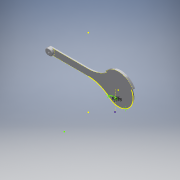
# Autodesk Inventor part: Trap
Saved by Autodesk Inventor 2019 (Build 230136000, 136)
## iProperties
Created: 2018-12-18
Part Number: Trap
Material: ABS Plastic
Document SubType Name: Modeling
Designer: assman
Density: 1.06 g/cm^3
Appearance: Smooth - White
Author: assman
Autodesk Inventor part; units mm, degrees
ref_plane "YZ Plane" through (0, 0, 0) normal (1, 0, 0) x (0, 1, 0)
ref_plane "XZ Plane" through (0, 0, 0) normal (0, 1, 0) x (-1, 0, 0)
ref_plane "XY Plane" through (0, 0, 0) normal (0, 0, 1) x (1, 0, 0)
sketch "Sketch1" plane through (0, 0, 0) normal (0, 0, 1) x (1, 0, 0)
  line L0 (-0.1193, 0) -> (89.8393, 0) construction
  line L1 (52.5778, -17.0836) -> (118.1369, -38.385) construction
  line L2 (85.3573, -27.7343) -> (99.4539, 15.6504) construction
  line L3 (-0.1193, 0) -> (89.8393, 0) construction
  circle A0 centre (-0.1193, 0) radius 89.8635 construction
  circle A1 centre (85.3573, -27.7343) radius 17.272 construction
  spline S0 degree 3 poles (0.7787, 2.3967) (0.465, 2.4986) (0.1311, 2.5381) (-0.1977, 2.5122) (-0.5266, 2.4864) (-0.8501, 2.3951) (-1.1441, 2.2453) (-1.438, 2.0956) (-1.702, 1.8874) (-1.9162, 1.6366) (-2.1305, 1.3858) (-2.2947, 1.0924) (-2.3967, 0.7787) (-2.4986, 0.465) (-2.5381, 0.1311) (-2.5122, -0.1977) (-2.4864, -0.5266) (-2.3951, -0.8501) (-2.2453, -1.1441) (-2.0956, -1.438) (-1.8874, -1.702) (-1.6366, -1.9162) (-1.3858, -2.1305) (-1.0924, -2.2947) (-0.7787, -2.3967) (-0.465, -2.4986) (-0.1311, -2.5381) (0.1977, -2.5122) (0.5266, -2.4864) (0.8501, -2.3951) (1.1441, -2.2453) (1.438, -2.0956) (1.702, -1.8874) (1.9162, -1.6366) (2.1305, -1.3858) (2.2947, -1.0924) (2.3967, -0.7787) (2.4986, -0.465) (2.5381, -0.1311) (2.5122, 0.1977) (2.4864, 0.5266) (2.3951, 0.8501) (2.2453, 1.1441) (2.0956, 1.438) (1.8874, 1.702) (1.6366, 1.9162) (1.3858, 2.1305) (1.0924, 2.2947) (0.7787, 2.3967) knots -1 -1 -1 -1 -0.9375 -0.9375 -0.9375 -0.875 -0.875 -0.875 -0.8125 -0.8125 -0.8125 -0.75 -0.75 -0.75 -0.6875 -0.6875 -0.6875 -0.625 -0.625 -0.625 -0.5625 -0.5625 -0.5625 -0.5 -0.5 -0.5 -0.4375 -0.4375 -0.4375 -0.375 -0.375 -0.375 -0.3125 -0.3125 -0.3125 -0.25 -0.25 -0.25 -0.1875 -0.1875 -0.1875 -0.125 -0.125 -0.125 -0.0625 -0.0625 -0.0625 0 0 0 0 construction
  line L4 (49.5282, -4.1632) -> (-0.9859, -4.1632)
  line L5 (-0.9859, 4.1632) -> (49.5282, 4.1632)
  line L6 (89.6474, 4.1685) -> (95.7232, 4.1685)
  arc A2 (-0.9859, 4.1632) -> (-0.9859, -4.1632) centre (-0.9859, 0) ccw
  arc A3 (49.5282, 4.1632) -> (77.0618, 14.5059) centre (49.5282, 45.9838) ccw
  arc A4 (77.0618, -14.5059) -> (49.5282, -4.1632) centre (49.5282, -45.9838) ccw
  arc A5 (77.0618, -14.5059) -> (77.0618, 14.5059) centre (89.75, 0) ccw
  circle A6 centre (-0.1193, 0) radius 107.8832 construction
  arc A7 (49.5282, 6.5241) -> (75.5075, 16.2829) centre (49.5282, 45.9838) ccw construction
  line L7 (49.5282, 6.5241) -> (-0.9859, 6.5241) construction
  arc A8 (-0.9859, 6.5241) -> (-0.9859, -6.5241) centre (-0.9859, 0) ccw construction
  line L8 (-0.9859, -6.5241) -> (49.5282, -6.5241) construction
  arc A9 (75.5075, -16.2829) -> (49.5282, -6.5241) centre (49.5282, -45.9838) ccw construction
  arc A10 (75.5075, -16.2829) -> (75.5075, 16.2829) centre (89.75, 0) ccw construction
  arc A11 (106.9656, 13.0998) -> (100.4733, 18.7881) centre (89.75, 0) ccw construction
  point P0 (118.1369, -38.385)
  point P1 (0.7787, 2.3967)
  dimension "d4" = 4.1632
  dimension "d25" = 41.8205
  constraints: 22 point on circle, 10 centre point, 10 end point, 4 tangent, 3 parallel, 2 coincident, 2 horizontal, 2 point on line, 1 concentric, 1 equal radius, 16 other
  measures "d4" radius of A2
  measures "d25" radius of A3
extrude "Extrusion1" add sketch "Sketch1" along normal blind 1.76
sketch "Sketch2" plane through (0, 0, 1.76) normal (0, 0, 1) x (1, 0, 0)
  line L0 (0, 0) -> (0, 4.1298) construction
  line L1 (0, 4.1298) -> (0, -2.9173) construction
  arc A0 (-0.9859, 4.1632) -> (-0.9859, -4.1632) centre (-0.9859, 0) ccw projected
  line L2 (49.5282, 4.1632) -> (-0.9859, 4.1632) projected
  line L3 (-0.9859, 4.1632) -> (0, 4.1632)
  line L4 (-0.9859, -4.1632) -> (49.5282, -4.1632) projected
  line L5 (-0.9859, -4.1632) -> (0, -4.1632)
  arc A1 (0.9859, -4.1632) -> (0.9859, 4.1632) centre (0.9859, 0) ccw
  line L6 (-49.5282, 4.1632) -> (0.9859, 4.1632)
  line L7 (0.9859, -4.1632) -> (-49.5282, -4.1632)
  spline S0 degree 3 poles (0.9023, 2.7771) (1.2658, 2.659) (1.6057, 2.4686) (1.8964, 2.2204) (2.187, 1.9721) (2.4282, 1.6662) (2.6017, 1.3257) (2.7753, 0.9851) (2.881, 0.6101) (2.911, 0.2291) (2.941, -0.1519) (2.8952, -0.5388) (2.7771, -0.9023) (2.659, -1.2658) (2.4686, -1.6057) (2.2204, -1.8964) (1.9721, -2.187) (1.6662, -2.4282) (1.3257, -2.6017) (0.9851, -2.7753) (0.6101, -2.881) (0.2291, -2.911) (-0.1519, -2.941) (-0.5388, -2.8952) (-0.9023, -2.7771) (-1.2658, -2.659) (-1.6057, -2.4686) (-1.8964, -2.2204) (-2.187, -1.9721) (-2.4282, -1.6662) (-2.6017, -1.3257) (-2.7753, -0.9851) (-2.881, -0.6101) (-2.911, -0.2291) (-2.941, 0.1519) (-2.8952, 0.5388) (-2.7771, 0.9023) (-2.659, 1.2658) (-2.4686, 1.6057) (-2.2204, 1.8964) (-1.9721, 2.187) (-1.6662, 2.4282) (-1.3257, 2.6017) (-0.9851, 2.7753) (-0.6101, 2.881) (-0.2291, 2.911) (0.1519, 2.941) (0.5388, 2.8952) (0.9023, 2.7771) knots -1 -1 -1 -1 -0.9375 -0.9375 -0.9375 -0.875 -0.875 -0.875 -0.8125 -0.8125 -0.8125 -0.75 -0.75 -0.75 -0.6875 -0.6875 -0.6875 -0.625 -0.625 -0.625 -0.5625 -0.5625 -0.5625 -0.5 -0.5 -0.5 -0.4375 -0.4375 -0.4375 -0.375 -0.375 -0.375 -0.3125 -0.3125 -0.3125 -0.25 -0.25 -0.25 -0.1875 -0.1875 -0.1875 -0.125 -0.125 -0.125 -0.0625 -0.0625 -0.0625 0 0 0 0 projected
  point P0 (0.9023, 2.7771)
  dimension "d8" = 4.1632
  dimension "d9" = 50.5141
  constraints: 10 end point, 5 horizontal alignment, 2 point on circle, 2 point on line, 1 centre point, 1 equal radius, 4 other
  measures "d8" radius of A0
  measures "d9" distance of L2.start L2.end
extrude "Extrusion2" cut sketch "Sketch2" against normal blind 1.76 contours S0
sketch "Sketch3" plane through (0, 0, 1.76) normal (0, 0, 1) x (1, 0, 0)
  spline S0 degree 3 poles (0.9023, 2.7771) (1.2658, 2.659) (1.6057, 2.4686) (1.8964, 2.2204) (2.187, 1.9721) (2.4282, 1.6662) (2.6017, 1.3257) (2.7753, 0.9851) (2.881, 0.6101) (2.911, 0.2291) (2.941, -0.1519) (2.8952, -0.5388) (2.7771, -0.9023) (2.659, -1.2658) (2.4686, -1.6057) (2.2204, -1.8964) (1.9721, -2.187) (1.6662, -2.4282) (1.3257, -2.6017) (0.9851, -2.7753) (0.6101, -2.881) (0.2291, -2.911) (-0.1519, -2.941) (-0.5388, -2.8952) (-0.9023, -2.7771) (-1.2658, -2.659) (-1.6057, -2.4686) (-1.8964, -2.2204) (-2.187, -1.9721) (-2.4282, -1.6662) (-2.6017, -1.3257) (-2.7753, -0.9851) (-2.881, -0.6101) (-2.911, -0.2291) (-2.941, 0.1519) (-2.8952, 0.5388) (-2.7771, 0.9023) (-2.659, 1.2658) (-2.4686, 1.6057) (-2.2204, 1.8964) (-1.9721, 2.187) (-1.6662, 2.4282) (-1.3257, 2.6017) (-0.9851, 2.7753) (-0.6101, 2.881) (-0.2291, 2.911) (0.1519, 2.941) (0.5388, 2.8952) (0.9023, 2.7771) knots -1 -1 -1 -1 -0.9375 -0.9375 -0.9375 -0.875 -0.875 -0.875 -0.8125 -0.8125 -0.8125 -0.75 -0.75 -0.75 -0.6875 -0.6875 -0.6875 -0.625 -0.625 -0.625 -0.5625 -0.5625 -0.5625 -0.5 -0.5 -0.5 -0.4375 -0.4375 -0.4375 -0.375 -0.375 -0.375 -0.3125 -0.3125 -0.3125 -0.25 -0.25 -0.25 -0.1875 -0.1875 -0.1875 -0.125 -0.125 -0.125 -0.0625 -0.0625 -0.0625 0 0 0 0 projected
  arc A0 (-0.9859, 4.1632) -> (-0.9859, -4.1632) centre (-0.9859, 0) ccw projected
  line L0 (0, 0) -> (0, 4.7549) construction
  line L1 (0, 4.7549) -> (0, -4.5684) construction
  arc A1 (-0.9859, 4.1632) -> (-0.9859, -4.1632) centre (-0.9859, 0) ccw construction
  line L2 (-0.9859, 4.1632) -> (0, 4.1632) construction
  line L3 (-0.9859, 4.1632) -> (49.5282, 4.1632) construction
  line L4 (-0.9859, -4.1632) -> (0, -4.1632) construction
  line L5 (49.5282, -4.1632) -> (-0.9859, -4.1632) construction
  arc A2 (0.9859, -4.1632) -> (0.9859, 4.1632) centre (0.9859, 0) ccw
  line L6 (0.9859, 4.1632) -> (0, 4.1632) construction
  line L7 (0.9859, -4.1632) -> (0, -4.1632) construction
  line L8 (0, 0) -> (-2.9199, 0) construction
  line L9 (-2.9199, 0) -> (2.9199, 0) construction
  line L10 (-0.9859, 4.1632) -> (0.9859, 4.1632)
  line L11 (-0.9859, -4.1632) -> (0.9859, -4.1632)
  dimension "d12" = 4.1632
  dimension "d13" = 0.9859
  constraints: 20 end point, 7 point on line, 3 point on circle, 3 symmetric about line, 1 centre point, 1 collinear, 1 horizontal, 1 tangent, 1 vertical, 3 other
  measures "d12" radius of A0
  measures "d13" distance of L2.start L2.end
extrude "Extrusion3" add sketch "Sketch3" along normal blind 2.0574
sketch "Sketch4" plane through (0, 0, 3.8174) normal (0, 0, 1) x (1, 0, 0)
  arc A0 (-0.9859, 4.1632) -> (-0.9859, -4.1632) centre (-0.9859, 0) ccw projected
  line L0 (0.9859, 4.1632) -> (-0.9859, 4.1632) projected
  arc A1 (0.9859, -4.1632) -> (0.9859, 4.1632) centre (0.9859, 0) ccw projected
  line L1 (-0.9859, -4.1632) -> (0.9859, -4.1632) projected
  point P0 (0, 0)
extrude "Extrusion4" add sketch "Sketch4" along normal blind 1
sketch "Sketch5" plane through (0, 0, 4.8174) normal (0, 0, 1) x (1, 0, 0)
  point P0 (0, 0)
  point P1 (0, 0)
  constraints: 1 other
hole "Hole1" at (0, 0, 4.8174) direction (0, 0, -1) diameter 2 depth 1
fillet "Fillet1" radius 1 4 edges at (0, 4.1632, 4.8174) (-5.1491, 0, 4.8174) (0, -4.1632, 4.8174) (5.1491, 0, 4.8174)
sketch "Sketch6" plane through (0, 0, 1.76) normal (0, 0, 1) x (1, 0, 0)
  point P0 (0, 0)
sketch "Sketch7" plane through (0, 0, 1.76) normal (0, 0, 1) x (1, 0, 0)
  circle A0 centre (0, 0) radius 1 construction
  circle A1 centre (0, 0) radius 109.0971 construction
  arc A2 (49.5282, 4.1632) -> (77.0618, 14.5059) centre (49.5282, 45.9838) ccw projected
  arc A3 (77.0618, -14.5059) -> (77.0618, 14.5059) centre (89.75, 0) ccw projected
  arc A4 (77.0618, -14.5059) -> (49.5282, -4.1632) centre (49.5282, -45.9838) ccw projected
  arc A5 (72.7976, 13.6695) -> (75.7451, 16.0112) centre (49.5282, 45.9838) ccw
  line L0 (72.7976, 13.6695) -> (73.9663, 12.0465)
  line L1 (108.6615, 9.7392) -> (106.8835, 8.8235)
  arc A6 (108.6615, 9.7392) -> (75.7451, 16.0112) centre (89.75, 0) ccw
  dimension "d27" = 2
  dimension "d28" = 21.272
  dimension "d29" = 1.623
  dimension "d30" = 0.9157
  constraints: 6 point on circle, 4 end point, 2 centre point, 2 line through centre, 1 coincident, 3 other
  measures "d27" radial gap between concentric circles of A2 A5
  measures "d28" radius of A6
  measures "d29" vertical distance of L0.start L0.end
  measures "d30" vertical distance of L1.start L1.end
extrude "Extrusion5" add sketch "Sketch7" against normal blind 3
sketch "Sketch9" plane through (0, 0, 1.76) normal (0, 0, 1) x (1, 0, 0)
  arc A0 (0.9859, -4.1632) -> (0.9859, 4.1632) centre (0.9859, 0) ccw construction
  line L0 (0.9859, -4.1632) -> (49.5282, -4.1632) construction
  arc A1 (77.0618, -14.5059) -> (49.5282, -4.1632) centre (49.5282, -45.9838) ccw construction
  arc A2 (77.0618, -14.5059) -> (106.8835, 8.8235) centre (89.75, 0) ccw construction
  line L1 (108.6615, 9.7392) -> (106.8835, 8.8235) construction
  arc A3 (108.6615, 9.7392) -> (75.7451, 16.0112) centre (89.75, 0) ccw construction
  arc A4 (72.7976, 13.6695) -> (75.7451, 16.0112) centre (49.5282, 45.9838) ccw construction
  line L2 (73.9663, 12.0465) -> (72.7976, 13.6695) construction
  arc A5 (49.5282, 4.1632) -> (73.9663, 12.0465) centre (49.5282, 45.9838) ccw construction
  line L3 (49.5282, 4.1632) -> (0.9859, 4.1632) construction
  line L4 (89.75, 0) -> (89.75, -25.8673) construction
  circle A6 centre (85.3573, -27.7343) radius 17.2734 construction
  line L5 (89.75, 0) -> (85.3573, -27.7343) construction
  circle A7 centre (87.7447, -12.6608) radius 2.0119 construction
  circle A8 centre (87.7447, -12.6608) radius 2.0119
  point P0 (0, 0)
  constraints: 4 end point, 2 centre point, 1 coincident, 1 point on line, 1 vertical
hole "Hole2" at (87.7447, -12.6608, 1.76) direction (0, 0, -1) diameter 2 end through all
body "Solid1"
